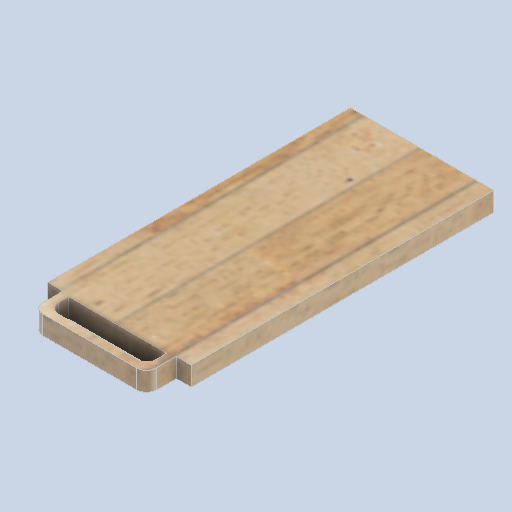
# Autodesk Inventor part: Part2
Saved by Autodesk Inventor 2022 (Build 260153000, 153)
## iProperties
Created: 2022-04-11
Part Number: Part2
Material: Wood (Maple)
Document SubType Name: Modeling
Designer: MacBook
Density: 0.67 g/cm^3
Appearance: Natural Maple - Glossy Dark Tint
Author: MacBook
Autodesk Inventor part; units mm, degrees
ref_plane "YZ Plane" through (0, 0, 0) normal (1, 0, 0) x (0, 1, 0)
ref_plane "XZ Plane" through (0, 0, 0) normal (0, 1, 0) x (-1, 0, 0)
ref_plane "XY Plane" through (0, 0, 0) normal (0, 0, 1) x (1, 0, 0)
sketch "Sketch1" plane through (0, 0, 0) normal (0, 1, 0) x (-1, 0, 0)
  line L0 (-72.2313, -152.4) -> (72.2313, -152.4)
  line L1 (72.2313, -152.4) -> (72.2312, 152.4)
  line L2 (72.2312, 152.4) -> (-72.2312, 152.4)
  line L3 (-72.2312, 152.4) -> (-72.2313, -152.4)
  line L4 (-72.2313, -152.4) -> (72.2312, 152.4) construction
  line L5 (72.2313, -152.4) -> (-72.2312, 152.4) construction
  point P0 (0, 0)
  dimension "d0" = 144.4625
  dimension "d1" = 304.8
  constraints: 12 end point, 2 midpoint, 2 parallel, 1 horizontal, 1 perpendicular
  measures "d0" distance between parallel lines of L3 L1
  measures "d1" distance between parallel lines of L0 L2
extrude "Extrusion1" add sketch "Sketch1" against normal blind 19.05
sketch "Sketch2" plane through (0, 0, 0) normal (0, 1, 0) x (1, 0, 0)
  line L0 (72.2312, -152.4) -> (-72.2312, -152.4) projected
  line L1 (-57.2312, -152.4) -> (57.2312, -152.4)
  line L2 (57.2312, -152.4) -> (57.2312, -182.4)
  line L3 (57.2312, -182.4) -> (-57.2312, -182.4)
  line L4 (-57.2312, -182.4) -> (-57.2312, -152.4)
  line L5 (-72.2313, 152.4) -> (-72.2312, -152.4) projected
  line L6 (72.2312, -152.4) -> (72.2313, 152.4) projected
  point P0 (0, 0)
  dimension "d4" = 15
  dimension "d5" = 15
  dimension "d6" = 30
  constraints: 8 end point, 2 parallel, 1 horizontal, 1 perpendicular, 1 point on line
  measures "d4" distance between parallel lines of L5 L4
  measures "d5" distance between parallel lines of L6 L2
  measures "d6" distance between parallel lines of L0 L3
extrude "Extrusion2" add sketch "Sketch2" against normal blind 19.05
sketch "Sketch3" plane through (0, 0, 0) normal (0, 1, 0) x (1, 0, 0)
  line L0 (-49.2312, -174.4) -> (49.2312, -174.4)
  line L1 (49.2312, -174.4) -> (49.2312, -154.4)
  line L2 (49.2312, -154.4) -> (-49.2312, -154.4)
  line L3 (-49.2312, -154.4) -> (-49.2312, -174.4)
  line L4 (-57.2312, -152.4) -> (-57.2312, -182.4) projected
  line L5 (-57.2312, -182.4) -> (57.2312, -182.4) projected
  line L6 (-72.2312, -152.4) -> (-57.2312, -152.4) projected
  line L7 (57.2312, -182.4) -> (57.2312, -152.4) projected
  point P0 (0, 0)
  point P1 (-57.2312, -167.4)
  dimension "d9" = 8
  dimension "d10" = 8
  dimension "d11" = 2
  dimension "d12" = 8
  constraints: 8 end point, 2 parallel, 1 horizontal, 1 midpoint, 1 perpendicular
  measures "d9" distance from line of point (-57.231, -167.4) L3
  measures "d10" distance between parallel lines of L5 L0
  measures "d11" distance between parallel lines of L6 L2
  measures "d12" distance between parallel lines of L7 L1
extrude "Extrusion3" cut sketch "Sketch3" against normal blind 19.05
fillet "Fillet1" radius 10 1 edges at (57.2312, -9.525, 182.4)
fillet "Fillet2" radius 10 1 edges at (-57.2312, -9.525, 182.4)
fillet "Fillet3" radius 10 1 edges at (-49.2312, -9.525, 174.4)
fillet "Fillet4" radius 10 1 edges at (49.2312, -9.525, 174.4)
body "Solid1"
